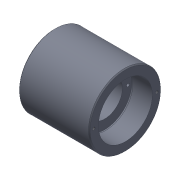
# Autodesk Inventor part: NA-45-h-Crown-187
Saved by Autodesk Inventor 2020.2 (Build 242310000, 310)
## iProperties
Created: 2020-09-21
Part Number: NA-45-h-Crown-187
Material: 19 436.4
Description: VODICI POUZDRO
Document SubType Name: Modeling
Designer: Jurek
Density: 7.85 g/cm^3
Appearance: RAL 7040 Window Grey(1)
Mass: 2004.69 g
Surface Area: 398.079 cm^2
Volume: 255.375 cm^3
User Status: Rozpracováno
Category: B
Hmotnost (kg): 2
Rozmer_A: 80
Rozmer_B: 0
Rozmer_C: 0
Rozmer_D: 78,5
Rada vyrobku: 4100
Prumer nadobky: 45
Cislo artiklu: 4451101322
C. variantniho vykresu: NA-45-h-Crown-187
Jednotka: ks
Cisty rozmer: =Ø<Rozmer_A> - <Rozmer_D>
Predpona: Ø
Stroj na lince: Stahovací lis
RAZ Poznamka 1: ISO 2768-mH
RAZ Poznamka 2: NEOZNAČENÉ HRANY OJEHLIT
DXF: Ne
QAD_code: M
Rizeni davek: L
Author: Správce
Revision Number: 00
Autodesk Inventor part; units mm, degrees
ref_plane "YZ Plane" through (0, 0, 0) normal (1, 0, 0) x (0, 1, 0)
ref_plane "XZ Plane" through (0, 0, 0) normal (0, 1, 0) x (-1, 0, 0)
ref_plane "XY Plane" through (0, 0, 0) normal (0, 0, 1) x (1, 0, 0)
sketch "Náčrt1" plane through (0, 0, 0) normal (0, 0, 1) x (1, 0, 0)
  line L0 (0, 0) -> (44.3557, 0)
  line L1 (0, 23) -> (0, 40)
  line L2 (0, 40) -> (78.5, 40)
  line L3 (78.5, 40) -> (78.5, 30)
  line L4 (78.5, 30) -> (56.9, 30)
  line L5 (55.5, 30) -> (55.5, 19.725)
  line L6 (55.5, 19.725) -> (11, 19.725)
  line L7 (11, 19.725) -> (11, 23)
  line L8 (9.6, 23) -> (0, 23)
  arc A0 (56.9, 30) -> (55.5, 30) centre (56.2, 28.875) ccw
  arc A1 (11, 23) -> (9.6, 23) centre (10.3, 21.875) ccw
  dimension "d0" = 80
  dimension "d1" = 46
  dimension "d2" = 11
  dimension "d6" = 78.5
  dimension "d7" = 60
  dimension "d8" = 23
  dimension "d9" = 39.45
  dimension "d27" = 0.2
  dimension "d28" = 1.4
  dimension "d31" = 0.2
  dimension "d32" = 1.4
  constraints: 18 end point, 6 parallel, 4 point on circle, 3 point on line, 2 centre point, 2 perpendicular, 1 horizontal
  measures "d0" diameter of L2 L0
  measures "d1" diameter of L8 L0
  measures "d2" distance between parallel lines of L7 L1
  measures "d6" distance between parallel lines of L3 L1
  measures "d7" diameter of L4 L0
  measures "d8" distance between parallel lines of L5 L3
  measures "d9" diameter of L6 L0
  measures "d27" distance edge to line of A1 L8
  measures "d28" distance from line of L8.start L7
  measures "d31" distance edge to line of A0 L4
  measures "d32" distance from line of L4.end L5
revolve "Rotace1" add sketch "Náčrt1" angle 360 about axis through (0, 0, 0) along (1, 0, 0)
chamfer "Zkosení1" distance 1 angle 45 2 edges at (78.5, -40, 0) (0, -40, 0)
chamfer "Zkosení2" distance 1 angle 30 1 edges at (0, -23, 0) measured on face at (0.5, -23, 0)
sketch "Náčrt2" plane through (0, 0, 0) normal (-1, 0, 0) x (0, 0, 1)
  circle A0 centre (0, 0) radius 26 construction
  point P0 (0, 26)
  point P1 (0, -26)
  dimension "d19" = 52
  constraints: 2 point on circle, 2 vertical alignment, 1 centre point, 1 coincident
  measures "d19" diameter of A0
hole "Díra1" at (0, 26, 0) at (0, -26, 0) direction (1, 0, 0) diameter 3.3 depth 55.5
sketch "Náčrt3" plane through (78.5, 0, 0) normal (1, 0, 0) x (0, 0, -1)
  circle A0 centre (0, 0) radius 35 construction
  point P0 (0, -35)
  point P1 (0, 35)
  dimension "d33" = 70
  constraints: 2 point on circle, 2 vertical alignment, 1 centre point, 1 coincident
  measures "d33" diameter of A0
hole "Díra2" at (78.5, -35, 0) at (78.5, 35, 0) direction (-1, 0, 0) diameter 3.242 depth 11.8 tip angle 118 thread size "M4x0.7" designation "M4" class "6H" standard "ISO Metric profile"
equation "\"Rozmer_B\" = 0"
equation "\"Rozmer_C\" = 0"
equation "\"Rozmer_D\" = d6"
